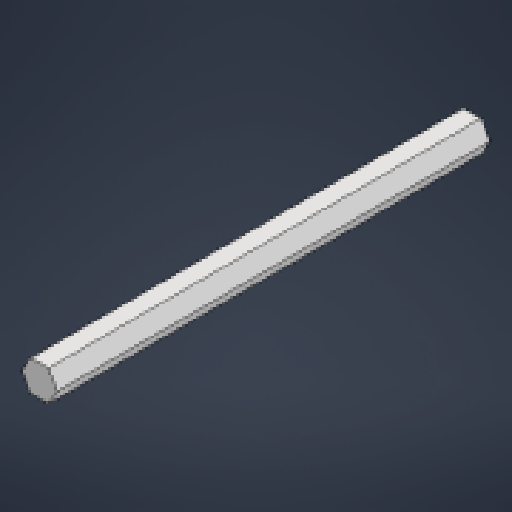
# Autodesk Inventor part: STOCK,HEX,SHAFT,VERTICAL
Saved by Autodesk Inventor 2026 (Build 300175000, 175)
## iProperties
Created: 2026-02-08
Part Number: STOCK,HEX,SHAFT,VERTICAL
Material: Generic
Document SubType Name: Modeling
Designer: littl
Density: 1 g/cm^3
Appearance: Default
Author: littl
Autodesk Inventor part; units mm, degrees
ref_plane "YZ Plane" through (0, 0, 0) normal (1, 0, 0) x (0, 1, 0)
ref_plane "XZ Plane" through (0, 0, 0) normal (0, 1, 0) x (-1, 0, 0)
ref_plane "XY Plane" through (0, 0, 0) normal (0, 0, 1) x (1, 0, 0)
sketch "Sketch1" plane through (0, 0, 0) normal (0, 0, 1) x (1, 0, 0)
  line L0 (3.6662, -6.35) -> (-3.6662, -6.35)
  line L1 (-3.6662, -6.35) -> (-7.3323, 0)
  line L2 (-7.3323, 0) -> (-3.6662, 6.35)
  line L3 (-3.6662, 6.35) -> (3.6662, 6.35)
  line L4 (3.6662, 6.35) -> (7.3323, 0)
  line L5 (7.3323, 0) -> (3.6662, -6.35)
  point P0 (0, 0)
  point P1 (0, 0)
  dimension "d0" = 12.7
  constraints: 12 end point, 1 coincident, 1 horizontal, 13 other
  measures "d0" distance between parallel lines of L3 L0
extrude "Extrusion1" add sketch "Sketch1" along normal blind 177.8
body "Solid1"
